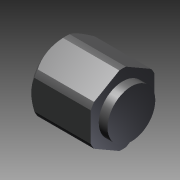
# Autodesk Inventor part: LWLF42...BCSNipple
Saved by Autodesk Inventor 2011 SP1 (Build 150282100, 282)
## iProperties
Created: 2015-04-20
Part Number: LWLF42...BCSNipple
Catalog Web Link: www.cadenas.de
Description: LWLF NIPPLE-LWLF
Vendor: IKO
Document SubType Name: Modeling
Designer: PARTuser1
Manufacturer: IKO
Mass: 0.0602039 g
Surface Area: 0.842015 cm^2
Volume: 0.0602039 cm^3
Density: 1 g/cm^3
Category: PARTsolutions
Company: IKO
Title: LWLF42...BCSNipple
Author: Cadenas PARTsolutions
Comments: LWLF
PSOL_IDENT_0: {$CADENAS_DATA\23d-libs\iko\linear_way_series\linear_way_l_series\lwlf\lwlf4\lwlf_nipple.prj},186 {V
PSOL_IDENT_1: TYP=3D},{NB=LWLF42...BCSNipple},{LINA=LWLF42...BCSNipple},{NN=LWLF NIPPLE},{DATE=29.01.2008 16:15:37
PSOL_IDENT_2: },{GEOMDATE=10.10.2007 11:14:00},{VERSION=},{LINEID=230},{LINESUBID=-1},{WBVAR=CP}  {NB=LWLF42...BCS
PSOL_IDENT_3: Nipple},{LINA=LWLF42...BCSNipple},{KT=DUMMY},{MNX=LWLF42...BCS},{H=16.00},{CP=},{Y=0.55},{VER=1.00}
SUPPLIER: IKO
ARTICLENO: LWLF42...BCSNipple
BOMINFO: LWLF42...BCSNipple
CREATOR: CADENAS GmbH
Autodesk Inventor part; units mm, degrees
sketch "Sketch_1" plane through (0, 0, 0) normal (0, 1, 0) x (-1, 0, 0)
  line L0 (0.9, 0) -> (5.2, 0)
  arc A0 (4.9894, -0.6) -> (5.2, 0) centre (4.24, 0) ccw
  arc A1 (4.0896, -2.2) -> (4.9894, -0.6) centre (2.05, 0) ccw
  line L1 (4.0896, -2.2) -> (0.9, -2.2)
  line L2 (0.9, -2.2) -> (0.9, -1.5)
  line L3 (0.9, -1.5) -> (-0.1, -1.5)
  line L4 (-0.1, -1.5) -> (-0.1, 0)
  line L5 (-0.1, 0) -> (5.2, 0)
  constraints: 12 end point, 4 point on circle, 2 centre point
revolve "Revolution1" add sketch "Sketch_1" angle 360 about axis through (-0.9, 0, 0) along (1, 0, 0)
sketch "Sketch_4" plane through (0, 0, 0) normal (0, 1, 0) x (-1, 0, 0)
  line L0 (-0.65, 0) -> (0.9, 0)
  line L1 (0.9, 0) -> (0.9, -2.2)
  line L2 (0.9, -2.2) -> (0.55, -2.2)
  line L3 (0.55, -2.2) -> (0.55, -1.5)
  line L4 (0.55, -1.5) -> (-0.65, -1.5)
  line L5 (-0.65, -1.5) -> (-0.65, 0)
  line L6 (-0.65, 0) -> (0.9, 0)
  constraints: 14 end point
revolve "Revolution2" add sketch "Sketch_4" angle 360 about axis through (0.65, 0, 0) along (1, 0, 0)
sketch "Sketch_2" plane through (0, 0, 0) normal (1, 0, 0) x (0, 1, 0)
  line L0 (4, 4.5) -> (-4, 4.5)
  line L1 (-4, 4.5) -> (-4, -4.5)
  line L2 (-4, -4.5) -> (4, -4.5)
  line L3 (4, -4.5) -> (4, 4.5)
  line L4 (0, 2.3094) -> (-2, 1.1547)
  line L5 (-2, 1.1547) -> (-2, -1.1547)
  line L6 (-2, -1.1547) -> (0, -2.3094)
  line L7 (0, -2.3094) -> (2, -1.1547)
  line L8 (2, -1.1547) -> (2, 1.1547)
  line L9 (2, 1.1547) -> (0, 2.3094)
  constraints: 20 end point
extrude "Extrusion1" cut sketch "Sketch_2" against normal blind 5
sketch "Sketch_9" plane through (0, 0, 0) normal (0, 1, 0) x (-1, 0, 0)
  line L0 (0, 8) -> (-5, 8)
  line L1 (-5, 8) -> (-5, -8)
  line L2 (-5, -8) -> (0, -8)
  line L3 (0, -8) -> (0, 8)
  constraints: 8 end point
extrude "Extrusion2" cut sketch "Sketch_9" along normal mid plane 36
ref_plane "4SLIDE_XY" through (0, 0, 0) normal (1, 0, 0) x (0, 0, -1)
ref_plane "4SLIDE_YZ" through (0, 0, 0) normal (0, 0, -1) x (0, 1, 0)
ref_plane "4SLIDE_ZX" through (0, 0, 0) normal (0, 1, 0) x (1, 0, 0)
body "Solid1"
